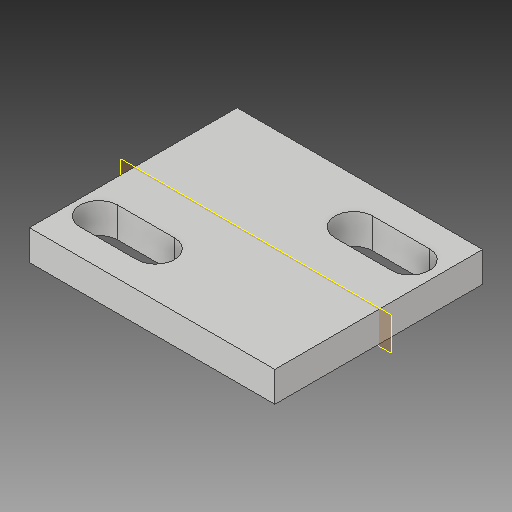
# Autodesk Inventor part: riser
Saved by Autodesk Inventor 2017 (Build 210142000, 142)
## iProperties
Created: 2018-12-03
Part Number: riser
Material: Generic
Document SubType Name: Modeling
Designer: Eric the Great
Density: 1 g/cm^3
Appearance: Default
Author: Eric the Great
Autodesk Inventor part; units mm, degrees
ref_plane "YZ Plane" through (0, 0, 0) normal (1, 0, 0) x (0, 1, 0)
ref_plane "XZ Plane" through (0, 0, 0) normal (0, 1, 0) x (-1, 0, 0)
ref_plane "XY Plane" through (0, 0, 0) normal (0, 0, 1) x (1, 0, 0)
sketch "Sketch1" plane through (0, 0, 0) normal (0, 1, 0) x (-1, 0, 0)
  line L0 (-13, 11) -> (13, 11)
  line L1 (13, 11) -> (13, -11)
  line L2 (13, -11) -> (-13, -11)
  line L3 (-13, -11) -> (-13, 11)
  line L4 (-13, 11) -> (13, -11) construction
  line L5 (13, 11) -> (-13, -11) construction
  line L6 (-4.1136, -6.25) -> (-10.1136, -6.25) construction
  line L7 (-4.1136, -4.25) -> (-10.1136, -4.25)
  line L8 (-10.1136, -8.25) -> (-4.1136, -8.25)
  arc A0 (-4.1136, -8.25) -> (-4.1136, -4.25) centre (-4.1136, -6.25) ccw
  arc A1 (-10.1136, -4.25) -> (-10.1136, -8.25) centre (-10.1136, -6.25) ccw
  line L9 (0, 0) -> (1.6306, 0)
  line L10 (10.3864, 6.25) -> (4.3864, 6.25) construction
  line L11 (10.3864, 8.25) -> (4.3864, 8.25)
  line L12 (4.3864, 4.25) -> (10.3864, 4.25)
  arc A2 (10.3864, 4.25) -> (10.3864, 8.25) centre (10.3864, 6.25) ccw
  arc A3 (4.3864, 8.25) -> (4.3864, 4.25) centre (4.3864, 6.25) ccw
  point P0 (-7.1136, -6.25)
  point P1 (7.3864, 6.25)
  dimension "d0" = 26
  dimension "d1" = 22
  dimension "d5" = 6
  dimension "d6" = 4
  dimension "d12" = 6
  dimension "d13" = 4
  dimension "d14" = 12.5
  dimension "d15" = 14.5
  constraints: 30 end point, 8 point on circle, 8 tangent, 4 centre point, 4 horizontal, 4 midpoint, 4 parallel, 1 perpendicular, 1 point on line, 1 other
  measures "d0" distance of L1.end L2.end
  measures "d1" distance of L0.end L1.end
  measures "d5" distance of L6.start L6.end
  measures "d6" distance between parallel lines of L8 L7
  measures "d12" distance of L10.start L10.end
  measures "d13" distance between parallel lines of L12 L11
  measures "d14" distance between parallel lines of L10 L6
  measures "d15" horizontal distance of point (-7.114, -6.25) point (7.386, 6.25)
extrude "Extrusion1" add sketch "Sketch1" along normal blind 3.2
ref_plane "Work Plane1" through (-13, 0, 0) normal (0, 0, 1) x (1, 0, 0)
body "Solid1"
